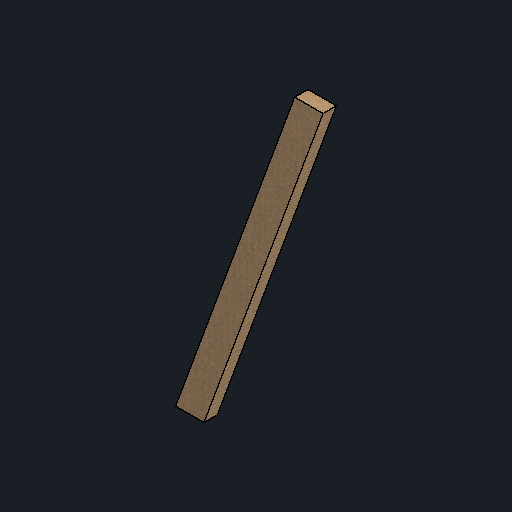
# Autodesk Inventor part: Part2
Saved by Autodesk Inventor 2026.2 (Build 302298000, 298)
## iProperties
Created: 2026-06-15
Part Number: Part2
Material: MDF Medium Density Fiberboard
Document SubType Name: Modeling
Designer: JoshuaEah
Density: 0.8 g/cm^3
Appearance: Cardboard - Corrugated
Author: JoshuaEah
Autodesk Inventor part; units mm, degrees
ref_plane "YZ Plane" through (0, 0, 0) normal (1, 0, 0) x (0, 1, 0)
ref_plane "XZ Plane" through (0, 0, 0) normal (0, 1, 0) x (-1, 0, 0)
ref_plane "XY Plane" through (0, 0, 0) normal (0, 0, 1) x (1, 0, 0)
sketch "Sketch1" plane through (0, 0, 0) normal (0, 0, 1) x (1, 0, 0)
  line L0 (0, 0) -> (0, 50.8)
  line L1 (0, 50.8) -> (104.2477, 337.2183)
  line L2 (0, 50.8) -> (304.8, 50.8) construction
  line L3 (104.2477, 337.2183) -> (304.8, 337.2183)
  line L4 (304.8, 337.2183) -> (304.8, 0)
  line L5 (304.8, 0) -> (0, 0)
  line L6 (1.7829, 0) -> (124.5203, 337.2183)
  line L7 (151.5504, 337.2183) -> (28.813, 0)
  line L8 (6.4053, 12.7) -> (33.4354, 12.7)
  line L9 (119.8979, 324.5183) -> (146.928, 324.5183)
  dimension "d0" = 50.8
  dimension "d1" = 304.8
  dimension "d2" = 70
  dimension "d6" = 304.8
  dimension "d7" = 19.05
  dimension "d8" = 25.4
  dimension "d9" = 12.7
  dimension "d10" = 12.7
  constraints: 20 end point, 8 point on line, 3 horizontal, 3 parallel, 2 perpendicular, 1 coincident, 1 equal length, 1 vertical
  measures "d0" distance of L0.start L0.end
  measures "d1" distance of L0.end L1.end
  measures "d2" angle of L2 L1
  measures "d6" distance of L4.end L0.start
  measures "d7" distance between parallel lines of L1 L6
  measures "d8" distance between parallel lines of L6 L7
  measures "d9" distance between parallel lines of L3 L9
  measures "d10" distance between parallel lines of L5 L8
extrude "Extrusion1" add sketch "Sketch1" along normal blind 12.7 contours L6 L9 L7 L8
body "Solid1"
